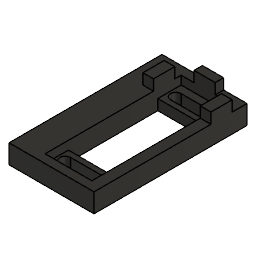
サーボモーター土台 (Autodesk Fusion 360 design; units mm, degrees)
Autodesk Fusion 360 part; units mm, degrees
note: some values were not read from the file. Set by a fixed rule: which sketch regions a step uses.
sketch "スケッチ1" plane through (0, 0, 0) normal (0, 0, 1) x (1, 0, 0)
  line L0 (0, 0) -> (22, 0)
  line L1 (22, 0) -> (22, 42)
  line L2 (22, 42) -> (0, 42)
  line L3 (0, 42) -> (0, 0)
  line L4 (-5, -15) -> (27, -15)
  line L5 (27, -15) -> (27, 57)
  line L6 (27, 57) -> (-5, 57)
  line L7 (-5, 57) -> (-5, -15)
  line L8 (1, 44.5) -> (21, 44.5)
  line L9 (21, 44.5) -> (21, 49.5)
  line L10 (21, 49.5) -> (1, 49.5)
  line L11 (1, 49.5) -> (1, 44.5)
  line L12 (1, 47) -> (21, 47)
  circle A0 centre (3.5, 47) radius 2.5
  circle A1 centre (18.5, 47) radius 2.5
  line L13 (22, 21) -> (-25, 21)
  line L14 (21, -7.5) -> (1, -7.5)
  line L15 (21, -2.5) -> (21, -7.5)
  circle A2 centre (18.5, -5) radius 2.5
  line L16 (1, -2.5) -> (21, -2.5)
  circle A3 centre (3.5, -5) radius 2.5
  line L17 (1, -5) -> (21, -5)
  line L18 (1, -7.5) -> (1, -2.5)
  dimension "d1" = 22
  dimension "d2" = 42
  dimension "d3" = 15
  dimension "d4" = 15
  dimension "d5" = 5
  dimension "d6" = 5
  dimension "d7" = 44.5
  dimension "d8" = 20
  dimension "d9" = 5
  dimension "d10" = 6
  dimension "d11" = 5
  dimension "d12" = 5
  constraint horizontal L0
  constraint vertical L1
  constraint horizontal L2
  constraint vertical L3
  constraint coincident L0.start L3.end
  constraint horizontal L4
  constraint vertical L5
  constraint horizontal L6
  constraint vertical L7
  constraint horizontal L8
  constraint vertical L9
  constraint horizontal L10
  constraint vertical L11
  constraint midpoint L11 L12.start
  constraint midpoint L9 L12.end
  constraint coincident L12 A0.centre
  constraint tangent L11 A0
  constraint coincident L12 A1.centre
  constraint tangent L9 A1
  constraint midpoint L1 L13.start
  constraint perpendicular L7 L13
  constraint symmetric L8.start L13 L16.start
  constraint symmetric L8.end L13 L15.start
  constraint symmetric L9.end L13 L14.start
  constraint symmetric L10.end L13 L14.end
  constraint symmetric L12.start L13 L17.start
  constraint symmetric L12.end L13 L17.end
  constraint symmetric A0 L13 A3
  constraint symmetric A1 L13 A2
  measures "d1" distance of L1.end L2.end
  measures "d2" distance of L0.start L2.end
  measures "d3" distance of L0 L4
  measures "d4" distance of L2 L6
  measures "d5" distance of L1 L5
  measures "d6" distance of L3 L7
  measures "d7" distance of L0 L8
  measures "d8" distance of L9.end L10.end
  measures "d9" distance of L8.end L9.end
  measures "d10" distance of L5 L9
  measures "d11" diameter of A0
  measures "d12" diameter of A1
extrude "押し出し1" add sketch "スケッチ1" along normal blind 5 contours L4 L5 L6 L7 | L8 L11 A0 | L10 L11 A0 | L8 L9 A1 | L9 L10 A1 | L14 L15 A2 | L15 A2 L16 | L14 A3 L18 | L16 A3 L18
sketch "スケッチ2" plane through (0, 0, 5) normal (0, 0, 1) x (-1, 0, 0)
  line L0 (0, 0) -> (0, -42)
  line L1 (0, -42) -> (-22, -42)
  line L2 (-22, -42) -> (-22, 0)
  line L3 (-22, 0) -> (0, 0)
  arc A0 (-18.5, -44.5) -> (-18.5, -49.5) centre (-18.5, -47) ccw
  line L4 (-18.5, -44.5) -> (-3.5, -44.5)
  arc A1 (-3.5, -49.5) -> (-3.5, -44.5) centre (-3.5, -47) ccw
  line L5 (-3.5, -49.5) -> (-18.5, -49.5)
  line L6 (5, -57) -> (5, 15)
  line L7 (5, 15) -> (-27, 15)
  line L8 (-27, 15) -> (-27, -57)
  line L9 (-27, -57) -> (5, -57)
  line L10 (5, -57) -> (-27, -57)
  line L11 (-27, -57) -> (-27, 15)
  line L12 (-27, 15) -> (5, 15)
  line L13 (5, 15) -> (5, -57)
  line L14 (0, -42) -> (-22, -42)
  line L15 (-22, -42) -> (-22, -53)
  line L16 (-22, -53) -> (0, -53)
  line L17 (0, -53) -> (0, -42)
  arc A2 (-18.5, 7.5) -> (-18.5, 2.5) centre (-18.5, 5) ccw
  line L18 (-18.5, 7.5) -> (-3.5, 7.5)
  arc A3 (-3.5, 2.5) -> (-3.5, 7.5) centre (-3.5, 5) ccw
  line L19 (-3.5, 2.5) -> (-18.5, 2.5)
  line L20 (-22, -21) -> (22.5657, -21)
  arc A4 (-3.5, 2.5) -> (-3.5, 7.5) centre (-3.5, 5) ccw
  line L21 (-18.5, 2.5) -> (-3.5, 2.5)
  line L22 (0, 0) -> (-22, 0)
  line L23 (0, 11) -> (0, 0)
  line L24 (-3.5, 7.5) -> (-18.5, 7.5)
  arc A5 (-18.5, 7.5) -> (-18.5, 2.5) centre (-18.5, 5) ccw
  line L25 (-22, 11) -> (0, 11)
  line L26 (-22, 0) -> (-22, 11)
  line L27 (0, 0) -> (-22, 0)
  constraint horizontal L10
  constraint vertical L11
  constraint horizontal L12
  constraint vertical L13
  constraint coincident L7.end L8.start
  constraint coincident L6.start L9.end
  constraint horizontal L14
  constraint vertical L15
  constraint horizontal L16
  constraint vertical L17
  constraint coincident L0.end L1.start
  constraint midpoint L2 L20.start
  constraint perpendicular L2 L20
  constraint symmetric L0.end L20 L0.start
  constraint symmetric L1.end L20 L2.end
  constraint symmetric A0.start L20 A2.end
  constraint symmetric A0.end L20 A2.start
  constraint symmetric A0 L20 A5
  constraint symmetric L4.end L20 A3.start
  constraint symmetric A1.start L20 L18.end
  constraint symmetric A1 L20 A4
  constraint symmetric L15.end L20 L25.start
  constraint symmetric L16.end L20 L23.start
extrude "押し出し2" add sketch "スケッチ2" along normal blind 4 contours L6 L7 L8 L9 L10 L11 L12 L13
sketch "スケッチ3" plane through (0, 0, 9) normal (0, 0, 1) x (-1, 0, 0)
  line L0 (-22, -53) -> (-22, 11)
  line L1 (0, 11) -> (0, -53)
  line L2 (0, -53) -> (-22, -53)
  line L3 (5, 15) -> (-27, 15)
  line L4 (-27, 15) -> (-27, -57)
  line L5 (-27, -57) -> (5, -57)
  line L6 (5, -57) -> (5, 15)
  line L7 (-16, -53) -> (-6, -53)
  line L8 (-6, -53) -> (-6, -57)
  line L9 (-6, -57) -> (-16, -57)
  line L10 (-16, -57) -> (-16, -53)
  line L11 (-22, 11) -> (0, 11)
  line L12 (-22, -50) -> (-27, -50)
  line L13 (-27, -50) -> (-27, -40)
  line L14 (-27, -40) -> (-22, -40)
  line L15 (-22, -40) -> (-22, -50)
  line L16 (0, -40) -> (5, -40)
  line L17 (5, -40) -> (5, -50)
  line L18 (5, -50) -> (0, -50)
  line L19 (0, -50) -> (0, -40)
  dimension "d17" = 11
  constraint horizontal L7
  constraint vertical L8
  constraint horizontal L9
  constraint vertical L10
  constraint coincident L5 L8.end
  constraint coincident L2 L7.start
  constraint horizontal L12
  constraint vertical L13
  constraint horizontal L14
  constraint vertical L15
  constraint coincident L4 L13.end
  constraint coincident L0 L12.start
  constraint horizontal L16
  constraint vertical L17
  constraint horizontal L18
  constraint vertical L19
  constraint coincident L1 L16.start
  measures "d17" distance of L4 L10
extrude "押し出し3" add sketch "スケッチ3" along normal blind 5 contours L0 L4 L12 L13 L14 L15 | L2 L5 L7 L8 L9 L10 | L1 L6 L16 L17 L18 L19
sketch "スケッチ5" plane through (-5, 0, 0) normal (-1, 0, 0) x (0, -1, 0)
  line L0 (-57, 0) -> (15, 0)
  line L1 (15, 0) -> (15, 9)
  line L2 (15, 9) -> (-40, 9)
  line L3 (-40, 9) -> (-40, 14)
  line L4 (-40, 14) -> (-50, 14)
  line L5 (-50, 14) -> (-50, 9)
  line L6 (-50, 9) -> (-57, 9)
  line L7 (-57, 9) -> (-57, 0)
  line L8 (15, 0) -> (-57, 0)
  line L9 (-57, 0) -> (-57, 9)
  line L10 (-57, 9) -> (15, 9)
  line L11 (15, 9) -> (15, 0)
  constraint horizontal L8
  constraint vertical L9
  constraint horizontal L10
  constraint vertical L11
  constraint coincident L6.end L7.start
  constraint coincident L0.end L1.start
extrude "押し出し5" add sketch "スケッチ5" along normal blind 8 contours L0 L1 L2 L6 L7 L8 L9 L10 L11
